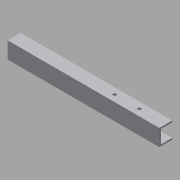
# Autodesk Inventor part: Firing Arm
Saved by Autodesk Inventor 2013 (Build 170138000, 138)
## iProperties
Created: 2013-01-08
Part Number: Firing Arm
Material: Aluminum 6061
Document SubType Name: Modeling
Designer: Naphat
Density: 2.71 g/cm^3
Mass: 341.078 g
Surface Area: 882.87 cm^2
Volume: 125.859 cm^3
Author: Naphat
Autodesk Inventor part; units mm, degrees
ref_plane "YZ Plane" through (0, 0, 0) normal (1, 0, 0) x (0, 1, 0)
ref_plane "XZ Plane" through (0, 0, 0) normal (0, 1, 0) x (-1, 0, 0)
ref_plane "XY Plane" through (0, 0, 0) normal (0, 0, 1) x (1, 0, 0)
sketch "Sketch1" plane through (0, 0, 0) normal (0, 0, 1) x (1, 0, 0)
  line L0 (-16, 12.5) -> (-13, 12.5)
  line L1 (-13, 12.5) -> (-13, -9.5)
  line L2 (-13, -9.5) -> (13, -9.5)
  line L3 (13, -9.5) -> (13, 12.5)
  line L4 (13, 12.5) -> (16, 12.5)
  line L5 (16, 12.5) -> (16, -12.5)
  line L6 (16, -12.5) -> (-16, -12.5)
  line L7 (-16, -12.5) -> (-16, 12.5)
  point P0 (0, 0)
  dimension "d0" = 3
  dimension "d2" = 3
  dimension "d3" = 25
  dimension "d4" = 32
  dimension "d5" = 16
  dimension "d7" = 12.5
  dimension "d8" = 3
  dimension "d74" = 25
  constraints: 16 end point, 5 parallel, 1 collinear, 1 horizontal, 1 perpendicular
  measures "d0" distance of L0.start L0.end
  measures "d2" distance of L3.end L4.end
  measures "d3" distance of L6.end L0.start
  measures "d4" distance of L5.end L6.end
  measures "d5" distance from line of point (0, 0) L7
  measures "d7" distance from line of L6 point (0, 0)
  measures "d8" distance between parallel lines of L6 L2
  measures "d74" distance between parallel lines of L6 L4
extrude "Extrusion1" add sketch "Sketch1" against normal blind 254
sketch "Sketch10" plane through (-16, -12.5, 0) normal (-1, 0, 0) x (0, 0, 1)
  line L0 (0, 0) -> (0, 25) projected
  line L1 (0, 25) -> (-254, 25) projected
  line L2 (0, 25) -> (-12.7, 25) construction
  line L3 (0, 25) -> (0, 12.5) construction
  line L4 (0, 12.5) -> (-12.7, 12.5) construction
  line L5 (-12.7, 12.5) -> (-60.325, 12.5) construction
  circle A0 centre (-12.7, 12.5) radius 3.175
  circle A1 centre (-60.325, 12.5) radius 3.175
  dimension "d134" = 12.7
  dimension "d136" = 12.5
  dimension "d138" = 47.625
  dimension "d139" = 6.35
  dimension "d140" = 6.35
  constraints: 8 end point, 2 centre point, 2 coincident, 2 collinear, 1 perpendicular, 1 point on line
  measures "d134" distance of L0.end L2.end
  measures "d136" distance of L0.end L3.end
  measures "d138" distance of L4.end L5.end
  measures "d139" diameter of A0
  measures "d140" diameter of A1
hole "Hole7" at (-16, 0, -12.7) at (-16, 0, -60.325) direction (1, 0, 0) diameter 6.35 depth 43 tip angle 118
sketch "Sketch11" plane through (0, 0, 0) normal (0, 0, 1) x (1, 0, 0)
  line L0 (-16, 12.5) -> (-13, 12.5) projected
  line L1 (-16, -12.5) -> (-16, 12.5) projected
  line L2 (16, -12.5) -> (-16, -12.5) projected
  line L3 (16, 12.5) -> (16, -12.5) projected
  line L4 (13, 12.5) -> (16, 12.5) projected
  line L5 (13, -9.5) -> (13, 12.5) projected
  line L6 (-13, -9.5) -> (13, -9.5) projected
  line L7 (-13, 12.5) -> (-13, -9.5) projected
  point P0 (0, 0)
extrude "Extrusion7" add sketch "Sketch11" along normal blind 38.1
equation "\"d2\" = d0"
equation "\"d5\" = 0.5 * d4"
equation "\"d7\" = 0.5 * d3"
equation "\"d8\" = d0"
equation "\"d74\" = d3"
equation "\"d140\" = d139"
body "Solid1"
